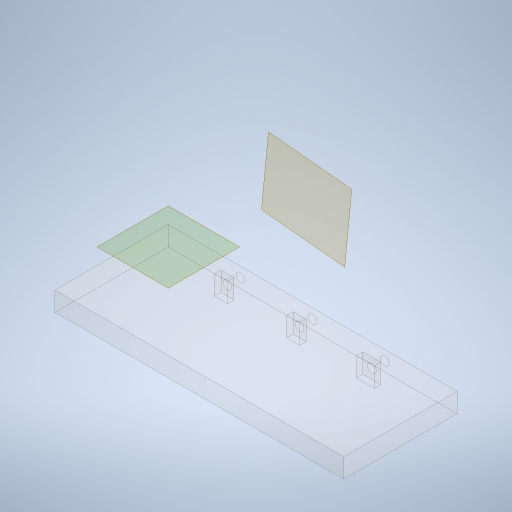
# Autodesk Inventor part: _head_adt_
Saved by Autodesk Inventor 2024.3 (Build 283343000, 343)
## iProperties
Created: 2024-09-08
Part Number: _head_adt_
Material: PMMA 플라스틱
Document SubType Name: Modeling
Designer: gretc
Density: 1.188 g/cm^3
Appearance: 폴리카보네이트 - 선명
Mass: 21.9535 g
Surface Area: 79.5521 cm^2
Volume: 18.4794 cm^3
Author: gretc
Autodesk Inventor part; units mm, degrees
ref_plane "YZ Plane" through (0, 0, 0) normal (1, 0, 0) x (0, 1, 0)
ref_plane "XZ Plane" through (0, 0, 0) normal (0, 1, 0) x (-1, 0, 0)
ref_plane "XY Plane" through (0, 0, 0) normal (0, 0, 1) x (1, 0, 0)
ref_plane "작업 평면4" through (-1.8693, 3.0801, 0) normal (0, 0, 1) x (0.9953009, -0.0968305, 0)
sketch "스케치1" plane through (-1.8693, 3.0801, 0) normal (0, 0, 1) x (0.9953009, -0.0968305, 0)
  circle A0 centre (-22.7477, 22.8243) radius 1.35 projected
  circle A1 centre (-43.8827, -21.2142) radius 1.35 projected
  circle A2 centre (21.6428, 27.143) radius 1.35 projected
  circle A3 centre (4.8701, -30.7532) radius 1.35 projected
  circle A4 centre (27.0653, -28.5939) radius 1.35 projected
  circle A5 centre (-0.5524, 24.9836) radius 1.35 projected
  circle A6 centre (-46.013, 0.6824) radius 1.3956 projected
  circle A7 centre (48.7397, 9.9006) radius 1.35 projected
  circle A8 centre (-17.3251, -32.9125) radius 1.35 projected
  circle A9 centre (50.8699, -11.996) radius 1.35 projected
  line L0 (68.8179, -26.0788) -> (63.0972, 32.7232) projected
  line L1 (60.913, 34.5202) -> (-62.7034, 22.4938) projected
  line L2 (-64.5004, 20.3096) -> (-58.7796, -38.4925) projected
  line L3 (-56.5954, -40.2895) -> (67.021, -28.2631) projected
  circle A10 centre (-49.3569, -21.7468) radius 1.35 projected
  circle A11 centre (-29.5905, 2.2801) radius 1.35 projected
  circle A12 centre (-51.4871, 0.1498) radius 1.35 projected
  circle A13 centre (-27.4602, -19.6165) radius 1.35 projected
  circle A14 centre (-38.4085, -20.6817) radius 1.35 projected
  circle A15 centre (-40.5388, 1.215) radius 1.35 projected
  circle A16 centre (34.4475, -13.5937) radius 1.35 projected
  circle A17 centre (54.2138, 10.4332) radius 1.35 projected
  circle A18 centre (45.3958, -12.5285) radius 1.35 projected
  circle A19 centre (32.3172, 8.3029) radius 1.35 projected
  circle A20 centre (43.2655, 9.3681) radius 1.35 projected
  circle A21 centre (56.3441, -11.4634) radius 1.35 projected
  circle A22 centre (-22.7477, 22.8243) radius 1.35 projected
  circle A23 centre (-43.8827, -21.2142) radius 1.35 projected
  circle A24 centre (21.6428, 27.143) radius 1.35 projected
  circle A25 centre (4.8701, -30.7532) radius 1.35 projected
  circle A26 centre (27.0653, -28.5939) radius 1.35 projected
  circle A27 centre (-0.5524, 24.9836) radius 1.35 projected
  circle A28 centre (-46.013, 0.6824) radius 1.3956 projected
  circle A29 centre (48.7397, 9.9006) radius 1.35 projected
  circle A30 centre (-17.3251, -32.9125) radius 1.35 projected
  circle A31 centre (50.8699, -11.996) radius 1.35 projected
  line L4 (68.8179, -26.0788) -> (63.0972, 32.7232) projected
  line L5 (-56.5954, -40.2895) -> (67.021, -28.2631) projected
  line L6 (-64.5004, 20.3096) -> (-58.7796, -38.4925) projected
  line L7 (60.913, 34.5202) -> (-62.7034, 22.4938) projected
  circle A32 centre (-49.3569, -21.7468) radius 1.35 projected
  circle A33 centre (-29.5905, 2.2801) radius 1.35 projected
  circle A34 centre (-51.4871, 0.1498) radius 1.35 projected
  circle A35 centre (-27.4602, -19.6165) radius 1.35 projected
  circle A36 centre (-38.4085, -20.6817) radius 1.35 projected
  circle A37 centre (-40.5388, 1.215) radius 1.35 projected
  circle A38 centre (34.4475, -13.5937) radius 1.35 projected
  circle A39 centre (54.2138, 10.4332) radius 1.35 projected
  circle A40 centre (45.3958, -12.5285) radius 1.35 projected
  circle A41 centre (32.3172, 8.3029) radius 1.35 projected
  circle A42 centre (43.2655, 9.3681) radius 1.35 projected
  circle A43 centre (56.3441, -11.4634) radius 1.35 projected
  line L8 (48.97, -23.4487) -> (-39.8109, -32.0859) projected
  line L9 (-39.8109, -32.0859) -> (-39.2299, -38.0578) projected
  line L10 (55.5228, -28.8395) -> (-45.2017, -38.6387) projected
  circle A44 centre (-17.3251, -32.9125) radius 1.35 projected
  circle A45 centre (4.8701, -30.7532) radius 1.35 projected
  circle A46 centre (27.0653, -28.5939) radius 1.35 projected
  line L11 (48.97, -23.4487) -> (-39.8109, -32.0859) projected
  line L12 (48.97, -23.4487) -> (49.551, -29.4205) projected
  circle A47 centre (-26.4824, -26.5694) radius 1.6 projected
  circle A48 centre (34.8281, -20.6047) radius 1.6 projected
  circle A49 centre (-30.5105, 14.8351) radius 1.6 projected
  circle A50 centre (30.8, 20.7999) radius 1.6 projected
  circle A51 centre (-26.4824, -26.5694) radius 1.6 projected
  circle A52 centre (34.8281, -20.6047) radius 1.6 projected
  circle A53 centre (-30.5105, 14.8351) radius 1.6 projected
  circle A54 centre (30.8, 20.7999) radius 1.6 projected
  arc A55 (67.021, -28.2631) -> (68.8179, -26.0788) centre (66.8273, -26.2725) ccw projected
  arc A56 (63.0972, 32.7232) -> (60.913, 34.5202) centre (61.1066, 32.5296) ccw projected
  arc A57 (-62.7034, 22.4938) -> (-64.5004, 20.3096) centre (-62.5098, 20.5032) ccw projected
  arc A58 (-58.7796, -38.4925) -> (-56.5954, -40.2895) centre (-56.789, -38.2989) ccw projected
  arc A59 (67.021, -28.2631) -> (68.8179, -26.0788) centre (66.8273, -26.2725) ccw projected
  arc A60 (-58.7796, -38.4925) -> (-56.5954, -40.2895) centre (-56.789, -38.2989) ccw projected
  arc A61 (-62.7034, 22.4938) -> (-64.5004, 20.3096) centre (-62.5098, 20.5032) ccw projected
  arc A62 (63.0972, 32.7232) -> (60.913, 34.5202) centre (61.1066, 32.5296) ccw projected
  point P0 (2.1588, -2.8846)
  point P1 (69.0116, -28.0694)
  point P2 (62.9036, 34.7138)
  point P3 (-64.694, 22.3002)
  point P4 (-58.586, -40.4831)
extrude "돌출1" add sketch "스케치1" along normal blind 35 contours L12 L10 L9 L8
sketch "스케치2" plane through (-1.8693, 3.0801, 35) normal (0, 0, 1) x (0.9953009, -0.0968305, 0)
  circle A0 centre (-17.3251, -32.9125) radius 1.35 projected
  circle A1 centre (4.8701, -30.7532) radius 1.35 projected
  circle A2 centre (27.0653, -28.5939) radius 1.35 projected
  point P0 (2.1588, -2.8846)
extrude "돌출2" add sketch "스케치2" against normal blind 30
ref_plane "작업 평면3" through (-44.6, -31.0001, 0) normal (0, -1, 0) x (1, 0, 0)
sketch "스케치3" plane through (-44.6, -31.0001, 0) normal (0, -1, 0) x (1, 0, 0)
  line L0 (45.95, 5) -> (43.25, 5) projected
  line L1 (68.25, 5) -> (65.55, 5) projected
  line L2 (23.65, 5) -> (20.95, 5) projected
  line L3 (64.0969, 4) -> (69.7031, 4)
  line L4 (69.7031, 4) -> (69.7031, 6)
  line L5 (69.7031, 6) -> (64.0969, 6)
  line L6 (64.0969, 6) -> (64.0969, 4)
  line L7 (64.0969, 4) -> (69.7031, 6) construction
  line L8 (69.7031, 4) -> (64.0969, 6) construction
  line L9 (42.6, 4) -> (46.6, 4)
  line L10 (46.6, 4) -> (46.6, 6)
  line L11 (46.6, 6) -> (42.6, 6)
  line L12 (42.6, 6) -> (42.6, 4)
  line L13 (42.6, 4) -> (46.6, 6) construction
  line L14 (46.6, 4) -> (42.6, 6) construction
  line L15 (20.3, 4) -> (24.3, 4)
  line L16 (24.3, 4) -> (24.3, 6)
  line L17 (24.3, 6) -> (20.3, 6)
  line L18 (20.3, 6) -> (20.3, 4)
  line L19 (20.3, 4) -> (24.3, 6) construction
  line L20 (24.3, 4) -> (20.3, 6) construction
  point P0 (44.6, 0)
  point P1 (66.9, 5)
  point P2 (44.6, 5)
  point P3 (22.3, 5)
  dimension "d4" = 2
  dimension "d5" = 4
  dimension "d6" = 2
  dimension "d7" = 4
  constraints: 36 end point, 9 midpoint, 6 parallel, 3 perpendicular, 1 horizontal
  measures "d4" distance of L4.end L3.end
  measures "d5" distance of L9.start L9.end
  measures "d6" distance of L10.end L9.end
  measures "d7" distance of L15.start L15.end
extrude "돌출4" cut sketch "스케치3" against normal up to surface (6 mm away)
